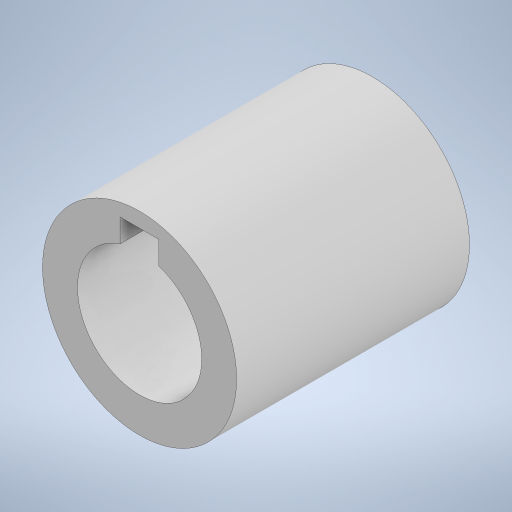
# Autodesk Inventor part: bearing_shaft_adapter
Saved by Autodesk Inventor 2023 (Build 270158000, 158)
## iProperties
Created: 2023-07-20
Part Number: bearing_shaft_adapter
Material: 一般
Document SubType Name: Modeling
Designer: 310611102
Density: 1 g/cm^3
Appearance: 預設
Author: 310611102
Autodesk Inventor part; units mm, degrees
ref_plane "YZ Plane" through (0, 0, 0) normal (1, 0, 0) x (0, 1, 0)
ref_plane "XZ Plane" through (0, 0, 0) normal (0, 1, 0) x (-1, 0, 0)
ref_plane "XY Plane" through (0, 0, 0) normal (0, 0, 1) x (1, 0, 0)
sketch "Sketch1" plane through (0, 0, 0) normal (0, 0, 1) x (1, 0, 0)
  circle A0 centre (0, 0) radius 12.5
  circle A1 centre (0, 0) radius 8
  line L0 (-2.5, 10.6) -> (2.5, 10.6)
  line L1 (2.5, 10.6) -> (2.5, 5.4)
  line L2 (2.5, 5.4) -> (-2.5, 5.4)
  line L3 (-2.5, 5.4) -> (-2.5, 10.6)
  line L4 (-2.5, 10.6) -> (2.5, 5.4) construction
  line L5 (2.5, 10.6) -> (-2.5, 5.4) construction
  point P0 (0, 8)
  point P1 (2.5, 7.5993)
  point P2 (-2.5, 7.5993)
  dimension "d0" = 16
  dimension "d1" = 25
  dimension "d2" = 2.6
  dimension "d3" = 5
  constraints: 12 end point, 2 coincident, 2 midpoint, 2 parallel, 1 centre point, 1 horizontal, 1 perpendicular, 1 vertical alignment, 3 other
  measures "d1" diameter of A0
  measures "d2" distance from line of point (0, 8) L0
  measures "d3" distance of L0.start L0.end
extrude "Extrusion1" add sketch "Sketch1" along normal blind 30
body "Solid1"
